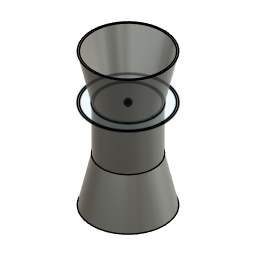
wzken爆改熔岩灯 (Autodesk Fusion 360 design; units mm, degrees)
Autodesk Fusion 360 part; units mm, degrees
sketch "草图1" plane through (0, 0, 0) normal (0, 1, 0) x (1, 0, 0)
  circle A0 centre (0, 0) radius 46.5
  circle A1 centre (0, 0) radius 33
  circle A2 centre (0, 0) radius 48.5
  circle A3 centre (0, 0) radius 35
  dimension "d1" = 93
  dimension "d2" = 66
  dimension "d3" = 97
  dimension "d4" = 70
  constraint coincident A0.centre A1.centre
  constraint concentric A0 A2
  constraint concentric A2 A3
  measures "d1" diameter of A0
  measures "d2" diameter of A1
  measures "d3" diameter of A2
  measures "d4" diameter of A3
extrude "拉伸3" add sketch "草图1" along normal blind 60 draft 12.7 contours A3
extrude "拉伸4" cut sketch "草图1" along normal blind 60 draft 12.7 contours A1
extrude "拉伸5" add sketch "草图1" against normal blind 60 contours A3
sketch "草图2" plane through (0, -60, 0) normal (0, -1, 0) x (1, 0, 0)
  circle A0 centre (0, 0) radius 33
  circle A1 centre (0, 0) radius 35
extrude "拉伸6" add sketch "草图2" along normal blind 60 draft 12.7
extrude "拉伸7" cut sketch "草图2" along normal blind 60 draft 12.7 contours A0
sketch "草图3" plane through (0, -120, 0) normal (0, -1, 0) x (1, 0, 0)
  circle A0 centre (0, 0) radius 46.5216
  circle A1 centre (0, 0) radius 48.5216
extrude "拉伸8" add sketch "草图3" against normal blind 2 draft 12.7 contours A0
